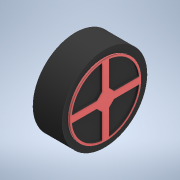
# Autodesk Inventor part: Part3proj
Saved by Autodesk Inventor 2020 (Build 240168000, 168)
## iProperties
Created: 2020-03-24
Part Number: Part3proj
Material: Rubber
Document SubType Name: Modeling
Designer: Manish
Density: 0.93 g/cm^3
Appearance: Rubber - Black
Author: Manish
Autodesk Inventor part; units mm, degrees
ref_plane "YZ Plane" through (0, 0, 0) normal (1, 0, 0) x (0, 1, 0)
ref_plane "XZ Plane" through (0, 0, 0) normal (0, 1, 0) x (-1, 0, 0)
ref_plane "XY Plane" through (0, 0, 0) normal (0, 0, 1) x (1, 0, 0)
sketch "Sketch1" plane through (0, 0, 0) normal (1, 0, 0) x (0, 1, 0)
  circle A0 centre (0, 0) radius 11
  dimension "d0" = 22
  constraints: 1 centre point, 1 coincident
  measures "d0" diameter of A0
extrude "Extrusion1" add sketch "Sketch1" along normal mid plane 10
sketch "Sketch2" plane through (-5, 0, 0) normal (-1, 0, 0) x (0, 0, 1)
  point P0 (0, 0)
sketch "Sketch3" plane through (0, 0, 0) normal (1, 0, 0) x (0, 1, 0)
  circle A0 centre (0, -0.2596) radius 13
  point P0 (0, 0)
  dimension "d3" = 26
  constraints: 1 centre point
  measures "d3" diameter of A0
extrude "Extrusion2" add sketch "Sketch3" along normal mid plane 9 separate body
hole "Hole1" at (-5, 0, 0) direction (1, 0, 0) diameter 2 depth 8 tip angle 118 bodies 1
sketch "Sketch4" plane through (-5, 0, 0) normal (-1, 0, 0) x (0, 0, 1)
  circle A0 centre (0, 0) radius 9.6784
  circle A1 centre (0, 0) radius 1 projected
  circle A2 centre (0, 0) radius 1.5
  dimension "d13" = 3
  constraints: 2 centre point, 2 coincident
  measures "d13" diameter of A2
extrude "Extrusion3" cut sketch "Sketch4" against normal blind 6 contours A0 bodies 1
sketch "Sketch6" plane through (5, 0, 0) normal (1, 0, 0) x (0, 0, -1)
  circle A0 centre (0, 0) radius 1.5 projected
  line L0 (-2.6563, -1.1003) -> (-2.6563, 1.1003)
  line L1 (-2.6563, 1.1003) -> (-1.1003, 2.6563)
  line L2 (-1.1003, 2.6563) -> (1.1003, 2.6563)
  line L3 (1.1003, 2.6563) -> (2.6563, 1.1003)
  line L4 (2.6563, 1.1003) -> (2.6563, -1.1003)
  line L5 (2.6563, -1.1003) -> (1.1003, -2.6563)
  line L6 (1.1003, -2.6563) -> (-1.1003, -2.6563)
  line L7 (-1.1003, -2.6563) -> (-2.6563, -1.1003)
  circle A1 centre (0, 0) radius 10.3309
  line L8 (-2.6563, -1.1003) -> (-10.2722, -1.1003)
  line L9 (-1.1003, 2.6563) -> (-1.1003, 10.2722)
  line L10 (2.6563, 1.1003) -> (10.2722, 1.1003)
  line L11 (1.1003, -2.6563) -> (1.1003, -10.2722)
  line L12 (-2.6563, 1.1003) -> (-10.2722, 1.1003)
  line L13 (-1.1003, -2.6563) -> (-1.1003, -10.2722)
  circle A2 centre (0, 0) radius 10.3309
  line L14 (2.6563, -1.1003) -> (10.2722, -1.1003)
  circle A3 centre (0, 0) radius 10.3309
  line L15 (1.1003, 2.6563) -> (1.1003, 10.2722)
  circle A4 centre (0, 0) radius 10.3309
  point P0 (1.1003, -10.2722)
  point P1 (10.2722, 1.1003)
  point P2 (-1.1003, 10.2722)
  dimension "d18" = 360
  dimension "d22" = 360
  constraints: 32 end point, 8 point on circle, 4 centre point, 4 coincident, 2 perpendicular, 1 horizontal, 61 other
extrude "Extrusion4" cut sketch "Sketch6" against normal through all contours L7 L13 A1 L8 | L12 A1 L9 L1 | L5 L14 A1 L11 | L15 A1 L10 L3 bodies 1
body "Solid1"
body "Solid2"
